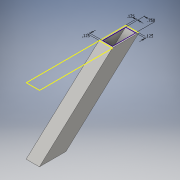
# Autodesk Inventor part: Diagonal Roller Cage Support
Saved by Autodesk Inventor 2016 (Build 200138000, 138)
## iProperties
Created: 2016-02-04
Part Number: Diagonal Roller Cage Support
Material: Generic
Document SubType Name: Modeling
Designer: gus
Density: 1 g/cm^3
Appearance: Default
Author: gus
Autodesk Inventor part; units mm, degrees
ref_plane "YZ Plane" through (0, 0, 0) normal (1, 0, 0) x (0, 1, 0)
ref_plane "XZ Plane" through (0, 0, 0) normal (0, 1, 0) x (-1, 0, 0)
ref_plane "XY Plane" through (0, 0, 0) normal (0, 0, 1) x (1, 0, 0)
sketch "Sketch3" plane through (0, 0, 0) normal (1, 0, 0) x (0, 1, 0)
  line L0 (0, 190.5) -> (127, 50.8)
  line L1 (0, 139.7) -> (127, 0)
  line L2 (127, 50.8) -> (127, 0)
  line L3 (0, 139.7) -> (0, 190.5)
  point P0 (0, 0)
  dimension "d10" = 34.1718
  dimension "d11" = 42.274
  dimension "d12" = 127
  constraints: 8 end point, 1 parallel, 1 vertical
  measures "d10" distance between parallel lines of L1 L0
  measures "d11" angle of L1 L2
  measures "d12" distance between parallel lines of L3 L2
extrude "Extrusion1" add sketch "Sketch3" along normal blind 25.4
sketch "Sketch4" plane through (0, 127, 50.8) normal (0, 1, 0) x (1, 0, 0)
  line L0 (0, -139.7) -> (0, 0) projected
  line L1 (25.4, 0) -> (25.4, -139.7) projected
  line L2 (0, 50.8) -> (25.4, 50.8) projected
  line L3 (0, -139.7) -> (25.4, -139.7) projected
  line L4 (22.225, 3.175) -> (3.175, 3.175)
  line L5 (3.175, 3.175) -> (3.175, 47.625)
  line L6 (3.175, 47.625) -> (22.225, 47.625)
  line L7 (22.225, 47.625) -> (22.225, 3.175)
  line L8 (0, 0) -> (0, 50.8) projected
  line L9 (0, 0) -> (25.4, 0) projected
  dimension "d19" = 3.175
  dimension "d20" = 3.175
  dimension "d21" = 3.175
  dimension "d22" = 19.05
  constraints: 8 end point, 2 parallel, 1 horizontal, 1 perpendicular
  measures "d19" distance between parallel lines of L5 L8
  measures "d20" distance between parallel lines of L6 L2
  measures "d21" distance between parallel lines of L9 L4
  measures "d22" distance of L5.end L6.end
sketch "Sketch6" plane through (0, 0, 139.7) normal (0, -1, 0) x (1, 0, 0)
  line L0 (22.225, 47.625) -> (3.175, 47.625)
  line L1 (3.175, 47.625) -> (3.175, 3.175)
  line L2 (3.175, 3.175) -> (22.225, 3.175)
  line L3 (22.225, 3.175) -> (22.225, 47.625)
  line L4 (25.4, 50.8) -> (25.4, 0) projected
  line L5 (0, 0) -> (25.4, 0) projected
  line L6 (0, 50.8) -> (25.4, 50.8) projected
  point P0 (0, -139.7)
  dimension "d27" = 19.05
  dimension "d28" = 3.175
  dimension "d29" = 3.175
  dimension "d30" = 3.175
  constraints: 8 end point, 2 parallel, 1 horizontal, 1 perpendicular
  measures "d27" distance of L1.end L2.end
  measures "d28" distance between parallel lines of L4 L3
  measures "d29" distance between parallel lines of L5 L2
  measures "d30" distance between parallel lines of L6 L0
sketch3d "3D Sketch1"
  line L0 (25.4, 0, 190.5) -> (25.4, 127, 50.8)
sweep "Sweep1" cut profiles "Sketch6" path "3D Sketch1"
equation "\"d28\" = d19"
equation "\"d29\" = d20"
equation "\"d30\" = d20"
body "Solid1"
